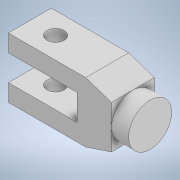
# Autodesk Inventor part: Schakel
Saved by Autodesk Inventor 2022 (Build 260153000, 153)
## iProperties
Created: 2022-06-01
Part Number: Schakel
Material: Generisch
Document SubType Name: Modeling
Designer: kaebi
Density: 1 g/cm^3
Appearance: Vorgabe
Author: kaebi
Autodesk Inventor part; units mm, degrees
ref_plane "YZ Plane" through (0, 0, 0) normal (1, 0, 0) x (0, 1, 0)
ref_plane "XZ Plane" through (0, 0, 0) normal (0, 1, 0) x (-1, 0, 0)
ref_plane "XY Plane" through (0, 0, 0) normal (0, 0, 1) x (1, 0, 0)
sketch "Skizze1" plane through (0, 0, 0) normal (0, 0, 1) x (1, 0, 0)
  line L0 (-3, 1.5) -> (5, 1.5)
  line L1 (-3, 1.5) -> (-3, 3.5)
  line L2 (-3, 3.5) -> (6, 3.5)
  line L3 (6, 3.5) -> (9, 2.5)
  line L4 (9, 2.5) -> (9, 0)
  line L5 (5, -1.5) -> (-3, -1.5)
  line L6 (-3, -1.5) -> (-3, -3.5)
  line L7 (-3, -3.5) -> (6, -3.5)
  line L8 (6, -3.5) -> (9, -2.5)
  line L9 (9, -2.5) -> (9, 0)
  line L10 (5, -1.5) -> (5, 1.5)
  point P0 (0, 0)
  point P1 (5, 0)
  dimension "d0" = 3
  dimension "d1" = 2
  dimension "d2" = 3
  dimension "d4" = 5
  dimension "d5" = 4
  dimension "d6" = 1
  dimension "d7" = 3
  constraints: 22 end point, 5 equal length, 4 perpendicular, 2 horizontal, 2 vertical, 2 vertical alignment, 1 horizontal alignment, 1 midpoint, 1 parallel
  measures "d0" distance between parallel lines of L0 L5
  measures "d1" distance of L0.start L1.end
  measures "d2" distance from line of point (0, 0) L1
  measures "d4" distance from line of point (0, 0) L10
  measures "d5" distance between parallel lines of L10 L4
  measures "d6" vertical distance of L2.end L3.end
  measures "d7" horizontal distance of L2.end L3.end
extrude "Extrusion1" add sketch "Skizze1" along normal mid plane 5
sketch "Skizze2" plane through (-3, 3.5, 2.5) normal (0, 1, 0) x (1, 0, 0)
  line L0 (3, 6) -> (3, -1) projected
  line L1 (14.4, 2.5) -> (-2.4, 2.5) projected
  circle A0 centre (3, 2.5) radius 1
  dimension "d10" = 2
  constraints: 1 centre point, 1 coincident
  measures "d10" diameter of A0
extrude "Extrusion2" cut sketch "Skizze2" along normal through all both and the other way through all
sketch "Skizze3" plane through (9, -2.5, 2.5) normal (1, 0, 0) x (0, 0, -1)
  circle A0 centre (2.5, 2.5) radius 2.5
  line L0 (5, 5) -> (5, 0) projected
  constraints: 1 centre point, 1 coincident, 1 tangent
extrude "Extrusion3" add sketch "Skizze3" along normal blind 2
